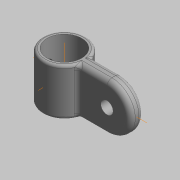
# Autodesk Inventor part: M50-5
Saved by Autodesk Inventor 2019.4 (Build 234330000, 330)
## iProperties
Created: 2020-04-23
Part Number: M50-5
Material: Generic
Document SubType Name: Modeling
Designer: Hannah
Density: 1 g/cm^3
Appearance: Default
Author: Hannah
Autodesk Inventor part; units mm, degrees
ref_plane "YZ Plane" through (0, 0, 0) normal (1, 0, 0) x (0, 1, 0)
ref_plane "XZ Plane" through (0, 0, 0) normal (0, 1, 0) x (-1, 0, 0)
ref_plane "XY Plane" through (0, 0, 0) normal (0, 0, 1) x (1, 0, 0)
sketch "Sketch2" plane through (0, 0, 0) normal (0, 1, 0) x (-1, 0, 0)
  circle A0 centre (0, 0) radius 14
  circle A1 centre (0, 0) radius 17.5
  dimension "d5" = 28
  dimension "d6" = 35
  constraints: 2 centre point, 2 coincident
  measures "d5" diameter of A0
  measures "d6" diameter of A1
extrude "Extrusion2" add sketch "Sketch2" along normal mid plane 38 contours A0 | A1
extrude "Extrusion3" cut sketch "Sketch2" along normal through all both and the other way through all contours A0
hole "Hole1" at (0, 0, 0) direction (-1, 0, 0) diameter 8.376 end through all thread size "M10x1.5" class "6H" standard "ISO Metric profile"
sketch "Sketch3" plane through (0, 0, 0) normal (0, 0, 1) x (1, 0, 0)
  circle A0 centre (40, 0) radius 5
  arc A1 (40, -19) -> (40, 19) centre (40, 0) ccw
  line L0 (14, 19) -> (40, 19)
  line L1 (40, -19) -> (14, -19)
  line L2 (0, -32.9) -> (0, 32.9) projected
  line L3 (14, -19) -> (14, 19) projected
  point P0 (0, 0)
  dimension "d36" = 10
  dimension "d37" = 19
  dimension "d40" = 40
  constraints: 4 end point, 2 centre point, 2 point on circle, 2 tangent, 1 coincident, 1 parallel
  measures "d36" diameter of A0
  measures "d37" radius of A1
  measures "d40" distance from line of L2 A0.centre
extrude "Extrusion5" add sketch "Sketch3" along normal mid plane 11
fillet "Fillet2" radius 4 6 edges at (59, 0, 5.5) (28.3066, -19, 5.5) (28.3066, 19, 5.5) (59, 0, -5.5) (28.3066, -19, -5.5) (28.3066, 19, -5.5)
fillet "Fillet2" radius 2 2 edges at (-17.5, 19, 0) (-17.5, -19, 0)
fillet "Fillet3" radius 4 12 edges at (16.6132, 0, 5.5) (16.6566, 16.0221, 5.3672) (16.439, 18.536, 3.3699) (-15.5, 19, 0) (16.4382, 18.537, -3.368) (16.6566, 16.0221, -5.3672) (16.6132, 0, -5.5) (16.6566, -16.0221, -5.3672) (16.467, -18.5015, -3.4338) (-15.5, -19, 0) (16.439, -18.536, 3.3699) (16.6566, -16.0221, 5.3672)
body "Solid1"
